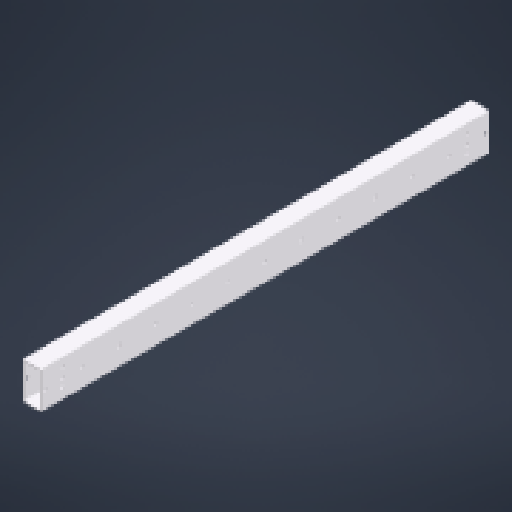
# Autodesk Inventor part: CRASH_BAR_INTAKE
Saved by Autodesk Inventor 2026.2 (Build 302298010, 298A)
## iProperties
Created: 2026-04-01
Part Number: CRASH_BAR_INTAKE
Material: Aluminum, 6061-T6
Document SubType Name: Modeling
Designer: 4aida
Density: 2.71 g/cm^3
Appearance: Metal-AL-6061 (Flat)
Mass: 392.355 g
Surface Area: 1836.28 cm^2
Volume: 144.78 cm^3
Author: 4aida
Autodesk Inventor part; units mm, degrees
ref_plane "YZ Plane" through (0, 0, 0) normal (1, 0, 0) x (0, 1, 0)
ref_plane "XZ Plane" through (0, 0, 0) normal (0, 1, 0) x (-1, 0, 0)
ref_plane "XY Plane" through (0, 0, 0) normal (0, 0, 1) x (1, 0, 0)
sketch "Sketch1" plane through (0, 0, 0) normal (0, 0, 1) x (1, 0, 0)
  line L0 (12.7, -25.4) -> (-12.7, -25.4)
  line L1 (-12.7, -25.4) -> (-12.7, 25.4)
  line L2 (-12.7, 25.4) -> (12.7, 25.4)
  line L3 (12.7, 25.4) -> (12.7, -25.4)
  line L4 (12.7, -25.4) -> (-12.7, 25.4) construction
  line L5 (-12.7, -25.4) -> (12.7, 25.4) construction
  line L6 (11.1125, -23.8125) -> (-11.1125, -23.8125)
  line L7 (-11.1125, -23.8125) -> (-11.1125, 23.8125)
  line L8 (-11.1125, 23.8125) -> (11.1125, 23.8125)
  line L9 (11.1125, 23.8125) -> (11.1125, -23.8125)
  line L10 (11.1125, -23.8125) -> (-11.1125, 23.8125) construction
  line L11 (-11.1125, -23.8125) -> (11.1125, 23.8125) construction
  point P0 (0, 0)
  dimension "d0" = 1.5875
  dimension "d1" = 1.5875
  dimension "d2" = 25.4
  dimension "d3" = 50.8
  constraints: 24 end point, 4 midpoint, 4 parallel, 2 horizontal, 2 perpendicular
  measures "d0" distance between parallel lines of L2 L8
  measures "d1" distance between parallel lines of L7 L1
  measures "d2" distance of L1.end L2.end
  measures "d3" distance of L0.end L1.end
extrude "Extrusion1" add sketch "Sketch1" along normal mid plane 622.3
sketch "Sketch2" plane through (12.7, -25.4, 311.15) normal (1, 0, 0) x (0, 0, -1)
  line L0 (0, 0) -> (0, 50.8) projected
  line L1 (0, 50.8) -> (622.3, 50.8) projected
  point P0 (311.15, 25.4)
  point P1 (5, 25.4)
  point P2 (30.4, 25.4)
  point P3 (0, 25.4)
  point P4 (30.4, 13.97)
  point P5 (30.4, 39.37)
  dimension "d6" = 25.4
  dimension "d7" = 5
  dimension "d30" = 11.43
  dimension "d31" = 25.4
  constraints: 2 horizontal alignment, 2 vertical alignment, 1 midpoint
  measures "d6" distance of point (5, 25.4) point (30.4, 25.4)
  measures "d7" distance from line of L0 point (5, 25.4)
  measures "d30" distance from line of L1 point (30.4, 39.37)
  measures "d31" distance of point (30.4, 13.97) point (30.4, 39.37)
hole "Hole1" at (12.7, 0, 306.15) at (12.7, 0, 280.75) at (12.7, 13.97, 280.75) at (12.7, -11.43, 280.75) direction (-1, 0, 0) diameter 5.105 end through all clearance for "Flat Head Machine Screw (82)" size "#10" standard "Ansi Unified Screw Threads"
mirror "Mirror1" about plane through (0, 0, 0) normal (0, 0, 1) of "Hole1"
sketch "Sketch3" plane through (12.7, -25.4, 311.15) normal (1, 0, 0) x (0, 0, -1)
  line L0 (622.3, 0) -> (0, 0) projected
  point P0 (311.15, 25.4)
  point P1 (311.15, 25.4)
  point P2 (260.35, 25.4)
  point P3 (209.55, 25.4)
  point P4 (158.75, 25.4)
  point P5 (107.95, 25.4)
  point P6 (57.15, 25.4)
  point P7 (361.95, 25.4)
  point P8 (311.15, 25.4)
  point P9 (260.35, 25.4)
  point P10 (209.55, 25.4)
  point P11 (158.75, 25.4)
  point P12 (107.95, 25.4)
  point P13 (412.75, 25.4)
  point P14 (361.95, 25.4)
  point P15 (311.15, 25.4)
  point P16 (260.35, 25.4)
  point P17 (209.55, 25.4)
  point P18 (158.75, 25.4)
  point P19 (463.55, 25.4)
  point P20 (412.75, 25.4)
  point P21 (361.95, 25.4)
  point P22 (311.15, 25.4)
  point P23 (260.35, 25.4)
  point P24 (209.55, 25.4)
  point P25 (514.35, 25.4)
  point P26 (463.55, 25.4)
  point P27 (412.75, 25.4)
  point P28 (361.95, 25.4)
  point P29 (311.15, 25.4)
  point P30 (260.35, 25.4)
  point P31 (565.15, 25.4)
  point P32 (514.35, 25.4)
  point P33 (463.55, 25.4)
  point P34 (412.75, 25.4)
  point P35 (361.95, 25.4)
  point P36 (311.15, 25.4)
  dimension "d17" = 50.8
  dimension "d20" = 50.8
  constraints: 2 horizontal, 1 coincident, 35 other
  measures "d17" distance of point (311.15, 25.4) point (260.35, 25.4)
  measures "d20" distance of point (311.15, 25.4) point (361.95, 25.4)
hole "Hole2" at (12.7, 0, 0) at (12.7, 0, 50.8) at (12.7, 0, 101.6) at (12.7, 0, 152.4) at (12.7, 0, 203.2) at (12.7, 0, 254) at (12.7, 0, -50.8) at (12.7, 0, -101.6) at (12.7, 0, -152.4) at (12.7, 0, -203.2) at (12.7, 0, -254) direction (-1, 0, 0) diameter 5.105 end through all clearance for "Flat Head Machine Screw (82)" size "#10" standard "Ansi Unified Screw Threads"
equation "\"d1\" = d0"
body "Solid1"
